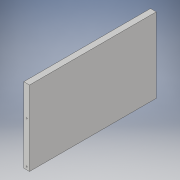
# Autodesk Inventor part: Cart Shelf
Saved by Autodesk Inventor 2018 (Build 220112000, 112)
## iProperties
Created: 2018-12-10
Part Number: Cart Shelf
Material: Generic
Document SubType Name: Modeling
Designer: Gabriel
Density: 1 g/cm^3
Appearance: Default
Author: Gabriel
Autodesk Inventor part; units mm, degrees
ref_plane "YZ Plane" through (0, 0, 0) normal (1, 0, 0) x (0, 1, 0)
ref_plane "XZ Plane" through (0, 0, 0) normal (0, 1, 0) x (-1, 0, 0)
ref_plane "XY Plane" through (0, 0, 0) normal (0, 0, 1) x (1, 0, 0)
sketch "Sketch2" plane through (0, 0, 0) normal (1, 0, 0) x (0, 1, 0)
  line L0 (32.64, 10.1333) -> (-297.56, 10.1333)
  line L1 (-297.56, 10.1333) -> (-297.56, -548.6667)
  line L2 (-297.56, -548.6667) -> (32.64, -548.6667)
  line L3 (32.64, -548.6667) -> (32.64, 10.1333)
  point P0 (0, 0)
  dimension "d0" = 330.2
  dimension "d1" = 558.8
  constraints: 8 end point, 2 parallel, 1 horizontal, 1 perpendicular
  measures "d0" distance of L2.end L1.end
  measures "d1" distance of L1.end L0.end
extrude "Extrusion2" add sketch "Sketch2" along normal blind 25.4
sketch "Sketch4" plane through (0, -297.56, -548.6667) normal (0, 0, -1) x (-1, 0, 0)
  line L0 (0, 0) -> (-25.4, 0) projected
  line L1 (-12.7, 0) -> (-12.7, 12.7)
  circle A0 centre (-12.7, 12.7) radius 2.5797
  line L2 (-12.7, 12.7) -> (-12.7, 196.5198)
  circle A1 centre (-12.7, 196.5198) radius 2.5797
  dimension "d25" = 12.7
  dimension "d26" = 5.1594
  dimension "d27" = 183.8198
  dimension "d28" = 5.1594
  constraints: 4 end point, 2 centre point, 2 coincident, 2 vertical, 1 midpoint
  measures "d25" distance of L1.start L1.end
  measures "d26" diameter of A0
  measures "d27" distance of L2.start L2.end
  measures "d28" diameter of A1
extrude "Extrusion4" cut sketch "Sketch4" against normal blind 914.4
body "Solid2"
